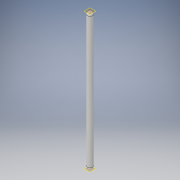
# Autodesk Inventor part: ball bearing replacement
Saved by Autodesk Inventor 2019 (Build 230136000, 136)
## iProperties
Created: 2020-01-28
Part Number: ball bearing replacement
Material: Generic
Document SubType Name: Modeling
Designer: User
Density: 1 g/cm^3
Appearance: Default
Author: User
Autodesk Inventor part; units mm, degrees
ref_plane "YZ Plane" through (0, 0, 0) normal (1, 0, 0) x (0, 1, 0)
ref_plane "XY Plane" through (0, 0, 0) normal (0, 0, 1) x (1, 0, 0)
sketch "Sketch1" plane through (0, 0, 0) normal (0, 1, 0) x (-1, 0, 0)
  circle A0 centre (0, 0) radius 1.6256
  dimension "d0" = 3.2512
  constraints: 1 centre point, 1 coincident
  measures "d0" diameter of A0
extrude "Extrusion1" add sketch "Sketch1" along normal blind 84.5058
fillet "Fillet1" radius 1.6256 2 edges at (1.6256, 84.5058, 0) (1.6256, 0, 0)
ref_plane "Work Plane1" through (0, 84.5058, 0) normal (0, 1, 0) x (-1, 0, 0)
body "Solid1"
